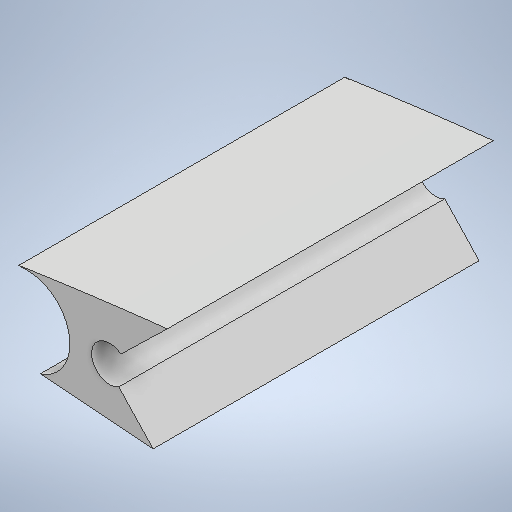
# Autodesk Inventor part: R10-11 Foam
Saved by Autodesk Inventor 2025.1 (Build 291241000, 241)
## iProperties
Created: 2024-10-23
Part Number: R10-11 Foam
Material: Generic
Document SubType Name: Modeling
Designer: 17jo6
Density: 1 g/cm^3
Appearance: Default
Author: 17jo6
Autodesk Inventor part; units mm, degrees
ref_plane "YZ Plane" through (0, 0, 0) normal (1, 0, 0) x (0, 1, 0)
ref_plane "XZ Plane" through (0, 0, 0) normal (0, 1, 0) x (-1, 0, 0)
ref_plane "XY Plane" through (0, 0, 0) normal (0, 0, 1) x (1, 0, 0)
sketch "Sketch1" plane through (0, 0, 0) normal (0, 0, 1) x (1, 0, 0)
  spline S0 degree 4 poles (254.4361, 38.2581) (252.1599, 38.6503) (246.7887, 39.4993) (237.9849, 40.6183) (225.3575, 41.7043) (211.2027, 42.3417) (196.3926, 42.4701) (181.0313, 42.0702) (165.5064, 41.2217) (149.7852, 40.0448) (134.1096, 38.5775) (118.6247, 36.8508) (103.5, 34.9393) (88.9016, 32.8834) (74.9958, 30.7382) (61.9178, 28.5627) (49.8271, 26.4098) (38.8354, 24.34) (29.0772, 22.4039) (20.6323, 20.6564) (13.6456, 19.1491) (6.9132, 17.6607) (2.9022, 16.74) (0.4691, 16.1882) (0, 16.065) knots 0.214297 0.214297 0.214297 0.214297 0.214297 0.24332 0.281775 0.321542 0.36238 0.404005 0.446178 0.488665 0.531231 0.573688 0.615803 0.657336 0.698047 0.737682 0.775986 0.812688 0.847495 0.880087 0.910093 0.937059 0.960363 1 1 1 1 1
  spline S1 degree 4 poles (300, 15.624) (299.8057, 13.313) (297.7085, 10.3432) (293.0509, 7.5008) (285.3959, 4.883) (278.1124, 3.2165) (269.5147, 1.8925) (259.681, 0.913) (248.7129, 0.2783) (236.7119, -0.0309) (223.8067, -0.0504) (210.1253, 0.1933) (195.7754, 0.645) (180.9677, 1.2494) (165.6517, 1.9825) (150.1916, 2.9048) (134.6873, 3.9451) (119.3375, 5.0495) (104.3042, 6.1987) (89.7566, 7.3561) (75.8492, 8.4887) (62.7429, 9.5824) (50.5811, 10.6226) (39.4971, 11.5797) (29.6294, 12.4513) (21.0712, 13.2264) (13.9639, 13.8721) (7.1036, 14.5126) (2.9683, 14.8997) (0.533, 15.1397) (-0.0042, 15.1841) knots 0 0 0 0 0 0.054372 0.079821 0.107912 0.138499 0.171341 0.206187 0.242784 0.280891 0.320277 0.360713 0.402023 0.443985 0.486373 0.528958 0.57146 0.613642 0.655265 0.696085 0.735853 0.774308 0.811174 0.846157 0.87893 0.909115 0.936252 0.959711 1 1 1 1 1
  arc A0 (0, 16.065) -> (-0.0042, 15.1841) centre (0.1158, 15.624) ccw
  line L0 (0.1158, 15.624) -> (227.9902, 15.624) construction
  line L1 (300, 15.624) -> (0.1158, 15.624) construction
  line L2 (300, 15.624) -> (200, 15.624) construction
  line L3 (200, 15.624) -> (200, 42.3773) construction
  line L4 (200, 15.624) -> (200, 0.5273)
  line L5 (0, 0) -> (0, 20.241)
  line L6 (0, 20.241) -> (238.581, 20.241) construction
  circle A1 centre (238.581, 20.241) radius 14
  line L7 (238.581, 20.241) -> (208.581, 20.241)
  line L8 (238.581, 25.359) -> (238.581, 20.241)
  line L9 (0, 20.241) -> (112, 20.241) construction
  line L10 (0, 15.624) -> (112, 15.624) construction
  line L11 (0, 15.624) -> (112, 15.624) construction
  line L12 (112, 15.624) -> (112, 35.9945)
  line L13 (112, 15.624) -> (112, 5.6153)
  spline S2 degree 4 poles (299.2852, 20.241) (299.2279, 20.1316) (299.168, 20.0232) (299.1056, 19.9158) (299.0406, 19.8092) knots 0.014818 0.014818 0.014818 0.014818 0.014818 0.017711 0.017711 0.017711 0.017711 0.017711
  line L14 (299.2071, 20.0822) -> (298.8742, 19.5363) construction
  arc A2 (298.904, 19.5932) -> (299.1702, 20.0296) centre (292.2911, 23.9254) ccw construction
  line L15 (299.432, 20.5214) -> (299.1384, 19.9606) construction
  arc A3 (299.1639, 20.0188) -> (299.3987, 20.4672) centre (292.801, 23.6361) ccw construction
  spline S3 degree 2 poles (295.8506, 16.56) (295.1573, 16.0692) (294.3933, 15.624) knots 0 0 0 1 1 1
  line L16 (294.5507, 15.7157) -> (294.2359, 15.5323) construction
  arc A4 (294.2672, 15.5511) -> (294.519, 15.6978) centre (283.8844, 33.657) ccw construction
  spline S4 degree 4 poles (296.8569, 15.624) (296.6183, 15.8629) (296.3707, 16.0985) (296.1147, 16.3309) (295.8506, 16.56) knots 0.044099 0.044099 0.044099 0.044099 0.044099 0.050856 0.050856 0.050856 0.050856 0.050856
  spline S5 degree 4 poles (219.5872, 34.9119) (218.6954, 34.952) (214.8585, 35.1063) (210.7072, 35.3295) (192.898, 35.4464) (181.4278, 35.0555) (165.1774, 34.1819) (149.5619, 33.1267) (133.8284, 31.3479) (128.2654, 31.0974) (123.3908, 30.59) knots 0 0 0 0 0 0.139244 0.23322 0.363937 0.509983 0.657115 0.798105 1 1 1 1 1
  line L17 (295.9593, 16.4657) -> (295.7419, 16.6543) construction
  arc A5 (295.9374, 16.4843) -> (295.7635, 16.6352) centre (281.8729, 0.4516) ccw construction
  line L18 (232.7438, 34.3645) -> (201.1936, 35.6815) construction
  arc A6 (229.5868, 34.4549) -> (204.3471, 35.5085) centre (136.3483, -1896.3245) ccw construction
  arc A7 (264.2661, 15.123) -> (264.3608, 15.624) centre (238.581, 20.241) ccw
  circle A8 centre (238.581, 20.241) radius 24
  circle A9 centre (112, 20.241) radius 15.39
  spline S6 degree 4 poles (300, 15.624) (300.2691, 17.9337) (298.7834, 21.2677) (294.6934, 24.9798) (287.5317, 28.9406) (280.4869, 31.8205) (271.481, 34.7182) (262.4868, 36.793) (257.7004, 37.6957) (254.4361, 38.2581) knots 0 0 0 0 0 0.247555 0.363857 0.49255 0.632996 0.778264 1 1 1 1 1
  line L19 (285.2945, 32.941) -> (223.5776, 43.5753) construction
  arc A10 (278.7224, 32.6349) -> (229.6682, 41.0872) centre (217.2184, -177.7386) ccw construction
  line L20 (285.2945, 32.941) -> (223.5776, 43.5753) construction
  arc A11 (278.8771, 33.0418) -> (229.6586, 41.5224) centre (200.8949, -272.4733) ccw construction
  spline S7 degree 4 poles (251.493, 31.7362) (243.7009, 32.9676) (232.1602, 34.2966) (216.4428, 35.2879) (196.3923, 35.4611) (181.0317, 35.0615) (165.5053, 34.2127) (149.7883, 33.0365) (134.1012, 31.5672) (118.6474, 29.8462) (103.4397, 27.9193) (89.0589, 25.9037) (74.8371, 23.6927) (62.4884, 21.6695) (49.6399, 19.3545) (46.3795, 18.7429) (43.8125, 18.259) knots 0 0 0 0 0 0.163963 0.232338 0.302031 0.372642 0.443778 0.515047 0.586134 0.656647 0.726187 0.794348 0.86071 0.920346 1 1 1 1 1 construction
  spline S8 degree 4 poles (295.845, 16.556) (295.7198, 16.6646) (294.585, 17.6283) (292.0585, 19.4283) (287.5167, 21.9347) (280.467, 24.8321) (271.9714, 27.5226) (264.2087, 29.4004) (258.4092, 30.5515) (255.0536, 31.1429) (254.4361, 31.2493) (253.9689, 31.3298) (253.5018, 31.4103) (253.0347, 31.4908) (252.5676, 31.5712) knots 0.050892 0.050892 0.050892 0.050892 0.050892 0.054094 0.079507 0.107628 0.138317 0.171335 0.206423 0.214297 0.214297 0.214297 0.214297 0.220253 0.220253 0.220253 0.220253 0.220253
  line L21 (285.2945, 25.9322) -> (223.5776, 36.5664) construction
  line L22 (285.2945, 25.9322) -> (223.5776, 36.5664) construction
  arc A12 (278.7224, 25.626) -> (229.6682, 34.0784) centre (217.2184, -184.7474) ccw construction
  line L23 (270.129, 9.1254) -> (275.129, 9.1254) construction
  line L24 (281.07, 24.4582) -> (286.07, 24.4582) construction
  line L25 (318.8214, -3.3673) -> (272.8686, 36.4793) construction
  arc A13 (303.2079, 0.552) -> (278.9595, 21.5782) centre (281.8576, 0.4252) ccw construction
  spline S9 degree 4 poles (295.8353, 16.5644) (293.4171, 14.8846) (288.4135, 12.6926) (280.7063, 10.6698) (269.511, 8.9398) (259.6826, 7.9632) (248.7122, 7.3273) (236.7121, 7.0186) (223.8065, 6.9989) (210.1254, 7.2427) (195.7753, 7.6944) (180.968, 8.2987) (165.6509, 9.032) (150.1939, 9.954) (134.681, 10.995) (119.3545, 12.0974) (104.259, 13.2519) (89.8748, 14.3954) (75.7524, 15.5471) (62.9065, 16.6165) (50.5107, 17.6776) (46.5166, 18.0246) (43.8125, 18.259) knots 0 0 0 0 0 0.084767 0.124025 0.166179 0.210904 0.257877 0.306788 0.35734 0.409241 0.462263 0.516122 0.570528 0.625186 0.679738 0.73388 0.787304 0.839697 0.89074 0.937143 1 1 1 1 1
  spline S10 degree 4 poles (21.4623, 20.241) (20.6227, 20.317) (20.124, 20.3622) (19.9191, 20.3809) (19.554, 20.414) knots 0.979732 0.979732 0.979732 0.979732 0.979732 1 1 1 1 1 construction
  line L26 (68.4884, 16.1198) -> (19.1367, 20.3983) construction
  arc A14 (63.5515, 16.5281) -> (24.0702, 19.9509) centre (-819.8994, -9944.3712) ccw construction
  line L27 (21.7244, 20.2173) -> (21.2001, 20.2647) construction
  arc A15 (21.2525, 20.26) -> (21.672, 20.222) centre (898.6358, 9712.9556) ccw construction
  line L28 (74.2541, 23.9969) -> (13.371, 12.5211) construction
  arc A16 (68.1759, 22.7939) -> (19.47, 13.6134) centre (1053.3901, -5337.891) ccw construction
  spline S11 degree 4 poles (218.4375, 7.1934) (217.6173, 7.2408) (213.8192, 7.4688) (209.5863, 6.8507) (192.5485, 7.9441) (181.1469, 8.163) (165.7461, 9.0283) (149.1424, 9.8801) (139.9777, 10.7519) (129.1073, 11.2464) (124.6867, 11.5289) knots 0 0 0 0 0 0.127631 0.213723 0.333628 0.467446 0.602621 0.738424 0.880395 0.880395 0.880395 0.880395 0.880395 construction
  line L29 (133.5337, 10.9635) -> (115.8396, 12.0942) construction
  arc A17 (117.618, 12.0789) -> (131.7678, 11.1747) centre (141.027, 267.2384) ccw construction
  line L30 (140.665, 32.3881) -> (106.1166, 28.792) construction
  arc A18 (137.222, 31.4497) -> (109.679, 28.5828) centre (140.6225, -134.9596) ccw construction
  circle A19 centre (238.581, 20.241) radius 18
  line L31 (238.581, 38.241) -> (225.78, 41.559)
  line L32 (238.581, 2.241) -> (224.22, 0)
  line L33 (214.581, 20.241) -> (214.581, 42.1266) construction
  line L34 (127.39, 20.241) -> (127.39, 11.5255) construction
  line L35 (127.39, 20.241) -> (131.3139, 20.241) construction
  line L36 (96.61, 20.241) -> (96.61, 13.8631) construction
  line L37 (270.129, 5.6153) -> (270.129, 15.624) construction
  line L38 (272.129, 7.6153) -> (272.129, 13.624)
  line L39 (268.129, 13.624) -> (268.129, 7.6153)
  arc A20 (268.129, 7.6153) -> (272.129, 7.6153) centre (270.129, 7.6153) ccw
  arc A21 (272.129, 13.624) -> (268.129, 13.624) centre (270.129, 13.624) ccw
  line L40 (270.129, 32.1807) -> (270.129, 22.172) construction
  line L41 (272.129, 30.1807) -> (272.129, 24.172)
  line L42 (268.129, 24.172) -> (268.129, 30.1807)
  arc A22 (272.129, 30.1807) -> (268.129, 30.1807) centre (270.129, 30.1807) ccw
  arc A23 (268.129, 24.172) -> (272.129, 24.172) centre (270.129, 24.172) ccw
  arc A24 (200, 42.3155) -> (199.8539, 42.3773) centre (190.581, 20.241) ccw
  arc A25 (171.273, 34.4958) -> (171.2681, 34.4892) centre (190.581, 20.241) ccw
  arc A26 (210.7484, 7.2304) -> (209.2875, 35.2765) centre (190.581, 20.241) ccw
  arc A27 (169.4455, 8.8703) -> (169.4744, 8.8168) centre (190.581, 20.241) ccw
  arc A28 (153.9768, 9.6824) -> (154.0303, 9.7394) centre (142.78, 20.241) ccw
  arc A29 (151.2419, 33.0959) -> (151.2193, 33.1107) centre (142.78, 20.241) ccw
  arc A30 (132.1299, 31.3508) -> (130.3229, 11.2037) centre (142.78, 20.241) ccw
  arc A31 (66.334, 16.3348) -> (66.5389, 15.624) centre (81.22, 20.241) ccw
  line L43 (112, 20.241) -> (112, 14.851) construction
  line L44 (112, 14.851) -> (91.265, 14.851) construction
  line L45 (112, 20.241) -> (87.265, 20.241) construction
  line L46 (87.265, 20.241) -> (87.265, 19.422) construction
  circle A32 centre (87.265, 19.422) radius 12.794
  line L47 (87.265, 32.216) -> (84.7014, 32.216)
  circle A33 centre (112.0123, 20.2492) radius 5.39
  line L48 (122.5954, 17.6185) -> (122.5954, 13.8685)
  line L49 (122.5954, 21.3685) -> (122.5954, 13.8685)
  line L50 (127.5954, 13.8685) -> (127.5954, 21.3685)
  line L51 (122.5954, 13.8685) -> (127.5954, 13.8685)
  line L52 (127.5954, 21.3685) -> (122.5954, 21.3685)
  line L53 (112.0123, 20.2492) -> (146.6953, 20.2492) construction
  line L54 (167.5954, 17.6185) -> (170.0954, 17.6185) construction
  line L55 (167.5954, 17.6185) -> (167.5954, 21.3685)
  line L56 (167.5954, 13.8685) -> (167.5954, 21.3685)
  line L57 (162.5954, 13.8685) -> (167.5954, 13.8685)
  line L58 (162.5954, 21.3685) -> (162.5954, 13.8685)
  line L59 (167.5954, 21.3685) -> (162.5954, 21.3685)
  line L60 (146.5954, 17.6185) -> (170.5954, 17.6185) construction
  line L61 (146.5954, 17.6185) -> (167.5954, 17.6185) construction
  arc A34 (179.5651, 35.2547) -> (178.1042, 7.2085) centre (198.2716, 20.2192) ccw
  line L62 (115.3793, 24.4582) -> (129.3538, 38.0195)
  line L63 (115.3793, 16.0238) -> (129.3538, 2.4625)
  line L64 (114.78, 15.624) -> (125.0954, 4.6416)
  point P0 (0.783, 16.254)
  point P1 (3.213, 16.812)
  point P2 (7.239, 17.724)
  point P3 (12.813, 18.96)
  point P4 (19.884, 20.484)
  point P5 (28.374, 22.245)
  point P6 (38.199, 24.195)
  point P7 (49.254, 26.28)
  point P8 (61.419, 28.446)
  point P9 (74.571, 30.636)
  point P10 (88.56, 32.793)
  point P11 (103.242, 34.86)
  point P12 (118.455, 36.783)
  point P13 (134.028, 38.511)
  point P14 (149.793, 39.984)
  point P15 (165.576, 41.16)
  point P16 (181.206, 41.985)
  point P17 (196.638, 42.363)
  point P18 (211.554, 42.222)
  point P19 (239.145, 40.389)
  point P20 (262.68, 36.666)
  point P21 (272.577, 34.218)
  point P22 (281.07, 31.467)
  point P23 (288.069, 28.491)
  point P24 (293.505, 25.359)
  point P25 (297.324, 22.137)
  point P26 (300, 15.624)
  point P27 (0.861, 15.105)
  point P28 (3.342, 14.868)
  point P29 (7.446, 14.481)
  point P30 (13.122, 13.953)
  point P31 (20.31, 13.296)
  point P32 (28.92, 12.519)
  point P33 (38.856, 11.64)
  point P34 (50.007, 10.674)
  point P35 (62.244, 9.63)
  point P36 (75.429, 8.529)
  point P37 (89.418, 7.389)
  point P38 (104.052, 6.228)
  point P39 (119.172, 5.076)
  point P40 (134.613, 3.966)
  point P41 (150.207, 2.928)
  point P42 (165.783, 2.013)
  point P43 (181.167, 1.263)
  point P44 (196.068, 0.663)
  point P45 (210.468, 0.225)
  point P46 (237.189, 0.039)
  point P47 (249.246, 0.378)
  point P48 (260.262, 1.05)
  point P49 (270.129, 2.076)
  point P50 (278.739, 3.462)
  point P51 (285.993, 5.211)
  point P52 (291.81, 7.314)
  point P53 (296.121, 9.756)
  point P54 (298.863, 12.531)
  point P55 (200, 15.624)
  point P56 (225.3642, 15.624)
  point P57 (238.581, 6.241)
  point P58 (238.581, 34.241)
  point P59 (225.3642, 15.624)
  point P60 (251.7978, 15.624)
  point P61 (0, 16.065)
  point P62 (0, 15.1838)
  point P63 (224.581, 20.241)
  point P64 (0, 9.065)
  point P65 (0.783, 9.254)
  point P66 (3.213, 9.812)
  point P67 (7.239, 10.724)
  point P68 (12.813, 11.96)
  point P69 (19.884, 13.484)
  point P70 (28.374, 15.245)
  point P71 (38.199, 17.195)
  point P72 (49.254, 19.28)
  point P73 (61.419, 21.446)
  point P74 (74.571, 23.636)
  point P75 (88.56, 25.793)
  point P76 (103.242, 27.86)
  point P77 (118.455, 29.783)
  point P78 (134.028, 31.511)
  point P79 (149.793, 32.984)
  point P80 (165.576, 34.16)
  point P81 (181.206, 34.985)
  point P82 (225.78, 34.559)
  point P83 (239.145, 33.389)
  point P84 (251.493, 31.745)
  point P85 (262.68, 29.666)
  point P86 (272.577, 27.218)
  point P87 (281.07, 24.467)
  point P88 (288.069, 21.491)
  point P89 (293.505, 18.359)
  point P90 (297.324, 15.137)
  point P91 (299.493, 11.879)
  point P92 (300, 8.624)
  point P93 (-0.0042, 22.1841)
  point P94 (0.861, 22.105)
  point P95 (3.342, 21.868)
  point P96 (7.446, 21.481)
  point P97 (13.122, 20.953)
  point P98 (20.31, 20.296)
  point P99 (28.92, 19.519)
  point P100 (38.856, 18.64)
  point P101 (50.007, 17.674)
  point P102 (62.244, 16.63)
  point P103 (75.429, 15.529)
  point P104 (89.418, 14.389)
  point P105 (104.052, 13.228)
  point P106 (119.172, 12.076)
  point P107 (134.613, 10.966)
  point P108 (150.207, 9.928)
  point P109 (165.783, 9.013)
  point P110 (181.167, 8.263)
  point P111 (196.068, 7.663)
  point P112 (210.468, 7.225)
  point P113 (224.22, 7)
  point P114 (237.189, 7.039)
  point P115 (249.246, 7.378)
  point P116 (260.262, 8.05)
  point P117 (270.129, 9.076)
  point P118 (278.739, 10.462)
  point P119 (285.993, 12.211)
  point P120 (291.81, 14.314)
  point P121 (296.121, 16.756)
  point P122 (298.863, 19.531)
  point P123 (300, 22.624)
  point P124 (18.7405, 20.241)
  point P125 (216.9687, 35.023)
  point P126 (0, 16.065)
  point P127 (296.8569, 15.624)
  point P128 (294.3933, 15.624)
  point P129 (219.5872, 34.9119)
  point P130 (123.3908, 30.59)
  point P131 (254.4361, 38.2581)
  point P132 (0, 9.0562)
  point P133 (0.783, 9.2452)
  point P134 (3.213, 9.8032)
  point P135 (7.239, 10.7152)
  point P136 (12.813, 11.9512)
  point P137 (19.884, 13.4752)
  point P138 (28.374, 15.2362)
  point P139 (38.199, 17.1862)
  point P140 (49.254, 19.2712)
  point P141 (61.419, 21.4372)
  point P142 (74.571, 23.6272)
  point P143 (88.56, 25.7842)
  point P144 (103.242, 27.8512)
  point P145 (118.455, 29.7742)
  point P146 (134.028, 31.5022)
  point P147 (149.793, 32.9752)
  point P148 (165.576, 34.1512)
  point P149 (181.206, 34.9762)
  point P150 (196.638, 35.3542)
  point P151 (211.554, 35.2132)
  point P152 (225.78, 34.5502)
  point P153 (262.68, 29.6572)
  point P154 (272.577, 27.2092)
  point P155 (297.324, 15.1282)
  point P156 (299.493, 11.8702)
  point P157 (300, 8.6152)
  point P158 (254.4361, 31.2493)
  point P159 (216.8848, -206.3625)
  point P160 (278.8769, 26.0734)
  point P161 (229.5906, 33.8662)
  point P162 (-0.0042, 22.2335)
  point P163 (0.861, 22.1544)
  point P164 (3.342, 21.9174)
  point P165 (7.446, 21.5304)
  point P166 (13.122, 21.0024)
  point P167 (28.92, 19.5684)
  point P168 (38.856, 18.6894)
  point P169 (50.007, 17.7234)
  point P170 (62.244, 16.6794)
  point P171 (75.429, 15.5784)
  point P172 (89.418, 14.4384)
  point P173 (104.052, 13.2774)
  point P174 (119.172, 12.1254)
  point P175 (134.613, 11.0154)
  point P176 (150.207, 9.9774)
  point P177 (165.783, 9.0624)
  point P178 (181.167, 8.3124)
  point P179 (196.068, 7.7124)
  point P180 (210.468, 7.2744)
  point P181 (224.22, 7.0494)
  point P182 (237.189, 7.0884)
  point P183 (249.246, 7.4274)
  point P184 (260.262, 8.0994)
  point P185 (278.739, 10.5114)
  point P186 (285.993, 12.2604)
  point P187 (296.121, 16.8054)
  point P188 (298.863, 19.5804)
  point P189 (300, 22.6734)
  point P190 (225.7, -0.0094)
  point P191 (252.2617, 0.522)
  point P192 (227.3495, 41.4508)
  point P193 (105.9778, 6.0782)
  point P194 (115.8008, 5.3277)
  point P195 (98.26, 27.1738)
  point P196 (260.4522, 30.1228)
  point P197 (123.5853, 30.3718)
  point P198 (134.5979, 31.5604)
  point P199 (134.4982, 31.5502)
  dimension "d63" = 25.588
  dimension "d17" = 100
  dimension "d19" = 20.241
  dimension "d20" = 238.581
  dimension "d21" = 28
  dimension "d37" = 112
  dimension "d39" = 112
  dimension "d40" = 0
  dimension "d43" = 10
  dimension "d55" = 4
  dimension "d56" = 90
  dimension "d58" = 4
  dimension "d59" = 20.735
  dimension "d61" = 24.735
  dimension "d62" = 0.819
  dimension "d64" = 34.683
  constraints: 133 end point, 63 point on circle, 34 centre point, 31 midpoint, 23 point on line, 9 horizontal, 8 perpendicular, 7 tangent, 5 symmetric about line, 3 coincident, 3 collinear, 1 parallel, 1 vertical, 206 other
  measures "d17" distance of L1.start L2.end
  measures "d19" distance of L5.start L5.end
  measures "d20" distance of L5.end L6.end
  measures "d21" diameter of A1
  measures "d37" distance of L5.end L9.end
  measures "d39" distance of L10.start L10.end
  measures "d40" distance between parallel lines of L11 L10
  measures "d43" radial gap between concentric circles of A1 A8
  measures "d55" radial gap between concentric circles of A1 A19
  measures "d56" angle of L34 L35
  measures "d58" diameter of A21
  measures "d59" distance of L43.end L44.end
  measures "d61" distance of L43.start L45.end
  measures "d62" distance of L45.end L46.end
  measures "d64" distance of L53.start L60.start
extrude "Extrusion3" add sketch "Sketch1" along normal blind 98 contours L62 A9 L12 S0 | L12 A9 A32 L47 S0 | L62 A33 L12 A9 | L12 A33 L13 S9 A32 A9 | A33 L64 S9 L13 | S9 L64 A9 S1 L13 | L13 S1 A9 A32 S9 | A9 S1 A32 | L64 S1 A9
body "Solid2"
